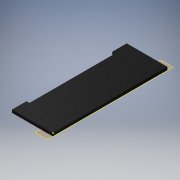
# Autodesk Inventor part: fronts
Saved by Autodesk Inventor 2018 (Build 220112000, 112)
## iProperties
Created: 2017-10-09
Part Number: fronts
Material: Generic
Document SubType Name: Modeling
Designer: HP
Density: 1 g/cm^3
Appearance: Fine Textured - Black
Author: HP
Autodesk Inventor part; units mm, degrees
ref_plane "YZ Plane" through (0, 0, 0) normal (1, 0, 0) x (0, 1, 0)
ref_plane "XZ Plane" through (0, 0, 0) normal (0, 1, 0) x (-1, 0, 0)
ref_plane "XY Plane" through (0, 0, 0) normal (0, 0, 1) x (1, 0, 0)
ref_plane "Work Plane1" through (0, 0, -5.5) normal (0, 0, 1) x (1, 0, 0)
sketch "Sketch1" plane through (0, 0, -5.5) normal (0, 0, 1) x (1, 0, 0)
  line L0 (0, 197) -> (0, 0) construction
  line L1 (0, 197) -> (-20, 197) construction
  line L2 (-20, 0) -> (-20, 197) construction
  line L3 (0, 0) -> (-20, 0) construction
  line L4 (0, -0.5) -> (-70, -0.5) construction
  line L5 (-70, -0.5) -> (-70, -5.5) construction
  line L6 (0, -5.5) -> (-70, -5.5) construction
  line L7 (0, -0.5) -> (0, -5.5) construction
  line L8 (-70, 197.5) -> (0, 197.5) construction
  line L9 (0, 197.5) -> (0, 202.5) construction
  line L10 (-70, 202.5) -> (0, 202.5) construction
  line L11 (-70, 197.5) -> (-70, 202.5) construction
  line L12 (0, -0.4) -> (0, 197.4)
  line L13 (0, -0.4) -> (-70, -0.4)
  line L14 (-70, -0.4) -> (-70, 24.5)
  line L15 (-70, 24.5) -> (-64.9, 24.5)
  line L16 (-64.9, 24.5) -> (-64.9, 172.5)
  line L17 (-64.9, 172.5) -> (-70, 172.5)
  line L18 (-70, 172.5) -> (-70, 197.4)
  line L19 (-70, 197.4) -> (0, 197.4)
  line L20 (-64.9, -0.5) -> (-64.9, -5.5) construction
  dimension "d1" = 0.1
  dimension "d2" = 0.1
  dimension "d3" = 24.9
  dimension "d4" = 24.9
  constraints: 16 end point, 6 perpendicular, 4 collinear, 1 point on line, 1 vertical
  measures "d1" distance from line of L12.start L4
  measures "d2" distance from line of L12.end L8
  measures "d3" distance between parallel lines of L15 L13
  measures "d4" distance between parallel lines of L17 L19
extrude "Extrusion1" add sketch "Sketch1" along normal blind 5
sketch "Sketch2" plane through (0, 0, -0.5) normal (0, 0, 1) x (1, 0, 0)
  point P0 (0, 0)
sketch "Sketch3" plane through (0, 0, -5.5) normal (0, 0, -1) x (-1, 0, 0)
  line L0 (0, 0) -> (0, 197) construction
  line L1 (0, 0) -> (20, 0) construction
  line L2 (20, 197) -> (20, 0) construction
  line L3 (0, 197) -> (20, 197) construction
  line L4 (10, 197) -> (10, 0) construction
  line L5 (0, -0.4) -> (0, 197.4) construction
  line L6 (0, 98.5) -> (20, 98.5) construction
  point P0 (10, 98.5)
  point P1 (10, 177)
  point P2 (10, 20)
  dimension "d7" = 20
  dimension "d8" = 20
  constraints: 5 midpoint, 4 end point, 2 point on line
  measures "d7" distance from line of point (10, 177) L3
  measures "d8" distance from line of point (10, 20) L1
hole "Hole1" at (-10, 98.5, -5.5) at (-10, 177, -5.5) at (-10, 20, -5.5) direction (0, 0, 1) diameter 5 end through all
sketch "Sketch4" plane through (-64.9, 24.5, -5.5) normal (-1, 0, 0) x (0, 0, 1)
  line L0 (0, 148) -> (0, 0) construction
  line L1 (0, 0) -> (5, 0) construction
  line L2 (5, 148) -> (5, 0) construction
  line L3 (0, 148) -> (5, 148) construction
  line L4 (2.5, 0) -> (2.5, 148) construction
  line L5 (5, 148) -> (5, 0) construction
  line L6 (5, 74) -> (0, 74) construction
  point P0 (5.5, -24.5)
  point P1 (2.5, 74)
  point P2 (2.5, 128)
  point P3 (2.5, 20)
  dimension "d16" = 20
  dimension "d17" = 20
  constraints: 5 midpoint, 4 end point, 2 point on line
  measures "d16" distance from line of point (2.5, 20) L1
  measures "d17" distance from line of point (2.5, 128) L3
hole "Hole2" at (-64.9, 98.5, -3) at (-64.9, 152.5, -3) at (-64.9, 44.5, -3) direction (1, 0, 0) diameter 2.459 depth 8.8 tip angle 118 thread size "M3x0.5" class "6H" standard "ISO Metric profile"
sketch "Sketch5" plane through (0, 0, -0.5) normal (0, 0, 1) x (1, 0, 0)
  line L0 (-56.1, 45.7295) -> (-64.9, 45.7295) construction
  line L1 (-56.1, 43.2705) -> (-64.9, 43.2705) construction
  line L2 (-56.1, 99.7295) -> (-64.9, 99.7295) construction
  line L3 (-56.1, 97.2705) -> (-64.9, 97.2705) construction
  line L4 (-56.1, 153.7295) -> (-64.9, 153.7295) construction
  line L5 (-56.1, 151.2705) -> (-64.9, 151.2705) construction
  line L6 (-64.9, 43.2705) -> (-64.9, 45.7295) construction
  line L7 (-64.9, 43.2705) -> (-64.9, 45.7295) construction
  line L8 (-64.9, 44.5) -> (-57.2589, 44.5) construction
  line L9 (-61.9, 41.65) -> (-58.9, 41.65)
  line L10 (-58.9, 41.65) -> (-58.9, 47.35)
  line L11 (-58.9, 47.35) -> (-61.9, 47.35)
  line L12 (-61.9, 47.35) -> (-61.9, 41.65)
  line L13 (-64.9, 151.2705) -> (-64.9, 153.7295) construction
  line L14 (-64.9, 151.2705) -> (-64.9, 153.7295) construction
  line L15 (-64.9, 152.5) -> (-56.2589, 152.5) construction
  line L16 (-61.9, 149.65) -> (-58.9, 149.65)
  line L17 (-58.9, 149.65) -> (-58.9, 155.35)
  line L18 (-58.9, 155.35) -> (-61.9, 155.35)
  line L19 (-61.9, 155.35) -> (-61.9, 149.65)
  line L20 (-64.9, 97.2705) -> (-64.9, 99.7295) construction
  line L21 (-64.9, 97.2705) -> (-64.9, 99.7295) construction
  line L22 (-64.9, 98.5) -> (-54.9007, 98.5) construction
  line L23 (-61.9, 95.65) -> (-58.9, 95.65)
  line L24 (-58.9, 95.65) -> (-58.9, 101.35)
  line L25 (-58.9, 101.35) -> (-61.9, 101.35)
  line L26 (-61.9, 101.35) -> (-61.9, 95.65)
  point P0 (0, 0)
  dimension "d25" = 5.7
  dimension "d26" = 3
  dimension "d27" = 3
  dimension "d28" = 5.7
  dimension "d29" = 3
  dimension "d30" = 3
  dimension "d31" = 5.7
  dimension "d32" = 3
  dimension "d33" = 3
  constraints: 40 end point, 9 equal length, 6 horizontal, 3 midpoint, 3 perpendicular, 3 other
  measures "d25" distance between parallel lines of L9 L11
  measures "d26" distance between parallel lines of L12 L6
  measures "d27" distance between parallel lines of L10 L12
  measures "d28" distance between parallel lines of L16 L18
  measures "d29" distance between parallel lines of L19 L13
  measures "d30" distance between parallel lines of L17 L19
  measures "d31" distance between parallel lines of L23 L25
  measures "d32" distance between parallel lines of L26 L20
  measures "d33" distance between parallel lines of L24 L26
extrude "Extrusion2" cut sketch "Sketch5" against normal through all
equation "\"d1\" = ABS_tolerance"
equation "\"d2\" = ABS_tolerance"
equation "\"d4\" = d3"
equation "\"d5\" = plate_thickness"
equation "\"d8\" = d7"
equation "\"d17\" = d16"
equation "\"plate_thickness\" = 5"
equation "\"basic_plate_offset\" = 0.5"
equation "\"ABS_tolerance\" = 0.1"
equation "\"laser_cutter_thickness\" = 0.1"
body "Solid1"
